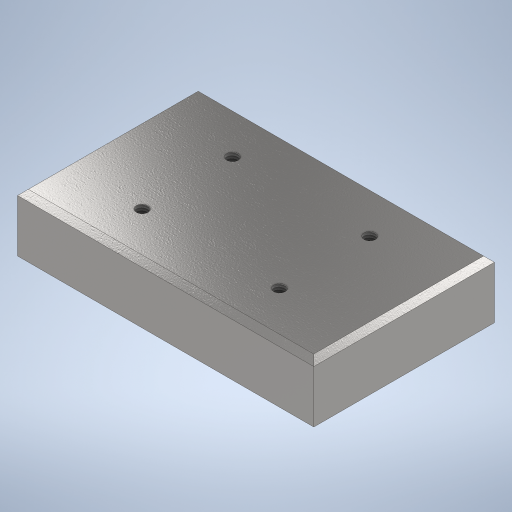
# Autodesk Inventor part: Grundplatte
Saved by Autodesk Inventor 2024 (Build 280153000, 153)
## iProperties
Created: 2024-01-15
Part Number: Grundplatte
Material: Stahl, galvanisiert
Document SubType Name: Modeling
Designer: ffogue
Density: 7.85 g/cm^3
Appearance: Galvanisiert
Author: ffogue
Autodesk Inventor part; units mm, degrees
ref_plane "YZ Plane" through (0, 0, 0) normal (1, 0, 0) x (0, 1, 0)
ref_plane "XZ Plane" through (0, 0, 0) normal (0, 1, 0) x (-1, 0, 0)
ref_plane "XY Plane" through (0, 0, 0) normal (0, 0, 1) x (1, 0, 0)
sketch "Skizze1" plane through (0, 0, 0) normal (0, 0, 1) x (1, 0, 0)
  line L0 (0, 50) -> (82, 50)
  line L1 (82, 50) -> (82, 0)
  line L2 (82, 0) -> (0, 0)
  line L3 (0, 0) -> (0, 50)
  dimension "d0" = 50
  dimension "d1" = 82
  constraints: 8 end point, 2 parallel, 1 coincident, 1 horizontal, 1 perpendicular
  measures "d0" distance between parallel lines of L2 L0
  measures "d1" distance between parallel lines of L1 L3
extrude "Extrusion1" add sketch "Skizze1" along normal blind 16
chamfer "Fasen1" distance 1.5 angle 45 4 edges at (41, 50, 16) (82, 25, 16) (41, 0, 16) (0, 25, 16)
sketch "Skizze2" plane through (0, 0, 16) normal (0, 0, 1) x (1, 0, 0)
  line L0 (82, 50) -> (0, 50) projected
  line L1 (41, 50) -> (41, 0) construction
  line L2 (0, 0) -> (82, 0) projected
  line L3 (0, 50) -> (0, 0) projected
  line L4 (0, 25) -> (82.1323, 25) construction
  point P0 (60, 37.5)
  point P1 (60, 12.5)
  point P2 (22, 37.5)
  point P3 (22, 12.5)
  dimension "d7" = 25
  dimension "d8" = 38
  constraints: 4 end point, 3 midpoint, 3 symmetric about line, 1 horizontal
  measures "d7" distance of point (60, 12.5) point (60, 37.5)
  measures "d8" distance of point (60, 37.5) point (22, 37.5)
hole "Bohrung1" at (60, 37.5, 16) at (60, 12.5, 16) at (22, 37.5, 16) at (22, 12.5, 16) direction (0, 0, -1) diameter 3.242 depth 8 tip angle 118 thread size "M4x0.7" class "6H" standard "ISO Metric profile"
